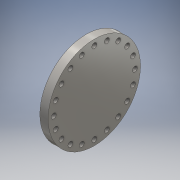
# Autodesk Inventor part: Blind Flange 14 in
Saved by Autodesk Inventor 2016 (Build 200138000, 138)
## iProperties
Created: 2018-11-05
Part Number: Blind Flange 14 in
Material: ASTM A105 Gr.B
Document SubType Name: Modeling
Designer: Wijaya
Mass: 106275 g
Surface Area: 7094.03 cm^2
Volume: 13538.2 cm^3
Density: 7.85 g/cm^3
Appearance: Semi-Polished
Author: Wijaya
Autodesk Inventor part; units mm, degrees
note: some values were not read from the file. Chosen so that the rebuilt part matches the saved one: direction of "Hole1".
ref_plane "YZ Plane" through (0, 0, 0) normal (1, 0, 0) x (0, 1, 0)
ref_plane "XZ Plane" through (0, 0, 0) normal (0, 1, 0) x (-1, 0, 0)
ref_plane "XY Plane" through (0, 0, 0) normal (0, 0, 1) x (1, 0, 0)
sketch "Sketch1" plane through (0, 0, 0) normal (0, 0, 1) x (1, 0, 0)
  line L0 (0, 0) -> (-284.4922, 0)
  line L1 (0, 0) -> (0, 292.5)
  line L2 (0, 292.5) -> (-52.4, 292.5)
  line L3 (-52.4, 292.5) -> (-52.4, 212.5)
  line L4 (-52.4, 212.5) -> (-54.4, 212.5)
  line L5 (-54.4, 212.5) -> (-54.4, 0)
  dimension "d0" = 585
  dimension "d1" = 52.4
  dimension "d2" = 2
  dimension "d3" = 425
  constraints: 12 end point, 4 perpendicular, 1 horizontal, 1 point on line, 1 vertical
  measures "d0" diameter of L2 L0
  measures "d1" distance of L1.end L2.end
  measures "d2" distance of L3.end L4.end
  measures "d3" diameter of L4 L0
revolve "Revolution1" add sketch "Sketch1" angle 360 about axis through (0, 0, 0) along (-1, 0, 0)
sketch "Sketch2" plane through (0, 0, 0) normal (1, 0, 0) x (0, 0, -1)
  point P0 (0, 0)
  point P1 (0, 257.2)
  dimension "d5" = 257.2
  constraints: 1 vertical alignment
  measures "d5" distance of point (0, 0) point (0, 257.2)
hole "Hole1" at (0, 257.2, 0) direction (-1, 0, 0) diameter 31.75 end up to surface
pattern_circular "Circular Pattern1" count 20 over 360 about axis through (-26.2, 0, 0) along (1, 0, 0) of "Hole1"
body "Solid1"
